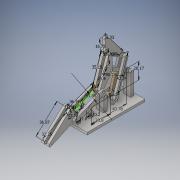
# Autodesk Inventor part: body
Saved by Autodesk Inventor 2016 (Build 200138000, 138)
## iProperties
Created: 2018-05-06
Part Number: body
Material: 一般
Document SubType Name: Modeling
Designer: 黃胤瑋
Density: 1 g/cm^3
Appearance: 預設
Author: 黃胤瑋
Autodesk Inventor part; units mm, degrees
ref_plane "YZ Plane" through (0, 0, 0) normal (1, 0, 0) x (0, 1, 0)
ref_plane "XZ Plane" through (0, 0, 0) normal (0, 1, 0) x (-1, 0, 0)
ref_plane "XY Plane" through (0, 0, 0) normal (0, 0, 1) x (1, 0, 0)
sketch "草圖1" plane through (0, 0, 0) normal (1, 0, 0) x (0, 1, 0)
  line L0 (0, 6) -> (-9.8716, 12.6095)
  line L1 (0, 18.8) -> (-17.0577, 32.3908)
  line L2 (-5.5713, 29.2426) -> (-17.0577, 32.3908)
  line L3 (-5.5713, 29.2426) -> (7.6738, 58.6472)
  line L4 (7.6738, 58.6472) -> (-17.0577, 32.3908)
  line L5 (-19.0401, -5.1652) -> (-52.4584, -16.0617)
  line L6 (-52.4584, -16.0617) -> (-35.2344, -17.5709)
  line L7 (-35.2344, -17.5709) -> (-19.0401, -5.1652)
  line L8 (-52.4584, -16.0617) -> (-69.1174, -14.5223)
  line L9 (-69.1174, -14.5223) -> (-40.2573, -36.5894)
  line L10 (-40.2573, -36.5894) -> (-52.4584, -16.0617)
  line L11 (-40.2573, -36.5894) -> (0, -23.8)
  line L12 (-19.0401, -5.1652) -> (-10.4, -10.2)
  line L13 (-35.2344, -17.5709) -> (-20.17, -43.78)
  line L14 (-19.0401, -5.1652) -> (-9.8716, 12.6095)
  line L15 (-5.5713, 29.2426) -> (-9.8716, 12.6095)
  line L16 (-5.5713, 29.2426) -> (-19.0401, -5.1652)
  point P0 (0, 0)
  dimension "d1" = 11.88
  dimension "d2" = 21.81
  dimension "d3" = 12.8
  dimension "d4" = 36.95
  dimension "d5" = 11.91
  dimension "d6" = 32.25
  dimension "d7" = 36.07
  dimension "d8" = 35.15
  dimension "d9" = 6
  dimension "d10" = 10.2
  dimension "d11" = 10.4
  dimension "d13" = 20.4
  dimension "d14" = 17.29
  dimension "d15" = 23.8
  dimension "d16" = 42.24
  dimension "d18" = 23.88
  dimension "d19" = 36.33
  dimension "d20" = 16.73
  dimension "d22" = 20.17
  dimension "d23" = 43.78
  dimension "d24" = 30.23
  dimension "d25" = 10
  dimension "d26" = 20
  dimension "d105" = 17.18
  constraints: 34 end point, 3 vertical alignment
  measures "d1" distance of L0.start L0.end
  measures "d2" distance of L1.end L1.start
  measures "d3" distance of L0.start L1.start
  measures "d4" distance of L5.start L2.start
  measures "d5" distance of L2.start L1.end
  measures "d6" distance of L2.start L3.end
  measures "d7" distance of L3.end L1.end
  measures "d8" distance of L5.start L5.end
  measures "d9" distance of point (0, 0) L0.start
  measures "d10" vertical distance of point (0, 0) L12.end
  measures "d11" horizontal distance of point (0, 0) L12.end
  measures "d13" distance of L6.end L5.start
  measures "d14" distance of L5.end L6.end
  measures "d15" distance of point (0, 0) L11.end
  measures "d16" distance of L9.end L11.end
  measures "d18" distance of L9.end L5.end
  measures "d19" distance of L8.end L9.end
  measures "d20" distance of L5.end L8.end
  measures "d22" horizontal distance of point (0, 0) L13.end
  measures "d23" vertical distance of point (0, 0) L13.end
  measures "d24" distance of L6.end L13.end
  measures "d25" distance of L5.start L12.end
  measures "d26" distance of L5.start L0.end
  measures "d105" distance of L2.start L0.end
sketch "草圖4" plane through (0, 0, 0) normal (1, 0, 0) x (0, 1, 0)
  line L0 (-53.0784, -14.1602) -> (-19.6601, -3.2637)
  line L1 (-17.8238, -6.7529) -> (-34.0182, -19.1586)
  line L2 (-35.409, -19.5633) -> (-52.633, -18.0541)
  arc A0 (-53.0784, -14.1602) -> (-52.633, -18.0541) centre (-52.4584, -16.0617) ccw
  arc A1 (-35.409, -19.5633) -> (-34.0182, -19.1586) centre (-35.2344, -17.5709) ccw
  arc A2 (-17.8238, -6.7529) -> (-19.6601, -3.2637) centre (-19.0401, -5.1652) ccw
  circle A3 centre (-19.0401, -5.1652) radius 1
  circle A4 centre (-52.4584, -16.0617) radius 1
  circle A5 centre (-35.2344, -17.5709) radius 1
  point P0 (0, 0)
  point P1 (-27.8274, -17.6895)
  dimension "d35" = 2
  dimension "d36" = 2
  dimension "d37" = 2
  dimension "d38" = 2
  constraints: 6 centre point, 6 coincident, 6 end point, 6 point on circle, 6 tangent, 2 equal radius
  measures "d35" radius of A0
  measures "d36" diameter of A3
  measures "d37" diameter of A4
  measures "d38" diameter of A5
extrude "擠出1" add sketch "草圖4" along normal mid plane 3
sketch "草圖5" plane through (-1.5, 0, 0) normal (-1, 0, 0) x (0, 0, 1)
  circle A0 centre (-5.1652, -19.0401) radius 1
  circle A1 centre (-10.2, -10.4) radius 1
  line L0 (-5.1652, -19.0401) -> (-10.2, -10.4) construction
  line L1 (-3.4372, -18.0331) -> (-8.472, -9.393)
  line L2 (-11.928, -11.407) -> (-6.8932, -20.047)
  arc A2 (-6.8932, -20.047) -> (-3.4372, -18.0331) centre (-5.1652, -19.0401) ccw
  arc A3 (-8.472, -9.393) -> (-11.928, -11.407) centre (-10.2, -10.4) ccw
  point P0 (0, 0)
  point P1 (-7.6826, -14.72)
  dimension "d41" = 2
  dimension "d42" = 2
  dimension "d43" = 1
  constraints: 8 end point, 4 centre point, 4 point on circle, 4 tangent, 2 coincident, 1 midpoint, 1 parallel
  measures "d41" diameter of A1
  measures "d42" diameter of A0
  measures "d43" radial gap between concentric circles of A1 A3
extrude "擠出2" add sketch "草圖5" along normal blind 3 separate body
sketch "草圖6" plane through (-1.5, 0, 0) normal (-1, 0, 0) x (0, 0, 1)
  line L0 (-17.5709, -35.2344) -> (-43.78, -20.17) construction
  line L1 (-16.5743, -33.5004) -> (-42.7833, -18.436)
  line L2 (-44.7767, -21.904) -> (-18.5676, -36.9684)
  arc A0 (-18.5676, -36.9684) -> (-16.5743, -33.5004) centre (-17.5709, -35.2344) ccw
  arc A1 (-42.7833, -18.436) -> (-44.7767, -21.904) centre (-43.78, -20.17) ccw
  circle A2 centre (-43.78, -20.17) radius 1
  circle A3 centre (-17.5709, -35.2344) radius 1
  point P0 (0, 0)
  point P1 (-30.6755, -27.7022)
  dimension "d46" = 2
  dimension "d47" = 2
  dimension "d48" = 1
  constraints: 8 end point, 4 centre point, 4 point on circle, 4 tangent, 2 coincident, 1 midpoint, 1 parallel
  measures "d46" diameter of A3
  measures "d47" diameter of A2
  measures "d48" radial gap between concentric circles of A2 A1
extrude "擠出3" add sketch "草圖6" along normal blind 3 separate body
sketch "草圖7" plane through (0, 0, 0) normal (1, 0, 0) x (0, 1, 0)
  circle A0 centre (0, -23.8) radius 1
  circle A1 centre (-40.2573, -36.5894) radius 1
  line L0 (-40.2573, -36.5894) -> (0, -23.8) construction
  line L1 (-40.8628, -34.6833) -> (-0.6056, -21.8939)
  line L2 (0.6056, -25.7061) -> (-39.6517, -38.4955)
  arc A2 (-40.8628, -34.6833) -> (-39.6517, -38.4955) centre (-40.2573, -36.5894) ccw
  arc A3 (0.6056, -25.7061) -> (-0.6056, -21.8939) centre (0, -23.8) ccw
  point P0 (0, 0)
  point P1 (-20.1286, -30.1947)
  dimension "d51" = 2
  dimension "d52" = 2
  dimension "d53" = 1
  constraints: 8 end point, 4 centre point, 4 point on circle, 4 tangent, 2 coincident, 1 midpoint, 1 parallel
  measures "d51" diameter of A0
  measures "d52" diameter of A1
  measures "d53" radial gap between concentric circles of A1 A2
extrude "擠出4" add sketch "草圖7" along normal mid plane 3 separate body
ref_plane "工作平面1" through (-3, 0, 0) normal (-1, 0, 0) x (0, 0, 1)
mirror "鏡射1" about plane through (-3, 0, 0) normal (-1, 0, 0) bodies 1 separate body
sketch "草圖8" plane through (-3, 0, 0) normal (-1, 0, 0) x (0, 0, 1)
  line L0 (-16.111, -70.3323) -> (-38.1782, -41.4721)
  line L1 (-35.5675, -38.538) -> (-15.0398, -50.7392)
  line L2 (-14.0702, -52.2744) -> (-12.5307, -68.9334)
  arc A0 (-16.111, -70.3323) -> (-12.5307, -68.9334) centre (-14.5223, -69.1174) ccw
  arc A1 (-14.0702, -52.2744) -> (-15.0398, -50.7392) centre (-16.0617, -52.4584) ccw
  arc A2 (-35.5675, -38.538) -> (-38.1782, -41.4721) centre (-36.5894, -40.2573) ccw
  circle A3 centre (-14.5223, -69.1174) radius 1
  circle A4 centre (-16.0617, -52.4584) radius 1
  circle A5 centre (-36.5894, -40.2573) radius 1 projected
  circle A6 centre (-36.5894, -40.2573) radius 1
  point P0 (0, 0)
  dimension "d57" = 2
  dimension "d58" = 2
  dimension "d59" = 2
  dimension "d60" = 2
  constraints: 6 centre point, 6 coincident, 6 end point, 6 point on circle, 6 tangent, 2 equal radius
  measures "d57" radius of A0
  measures "d58" diameter of A6
  measures "d59" diameter of A3
  measures "d60" diameter of A4
extrude "擠出5" add sketch "草圖8" along normal mid plane 3 separate body
mirror "鏡射2" about plane through (-3, 0, 0) normal (-1, 0, 0) bodies 4 separate body
sketch "草圖12" plane through (-1.5, 0, 0) normal (-1, 0, 0) x (0, 0, 1)
  circle A0 centre (6, 0) radius 1
  circle A1 centre (12.6095, -9.8716) radius 1
  line L0 (12.6095, -9.8716) -> (6, 0) construction
  line L1 (14.2714, -8.7589) -> (7.6619, 1.1127)
  line L2 (4.3381, -1.1127) -> (10.9476, -10.9843)
  arc A2 (10.9476, -10.9843) -> (14.2714, -8.7589) centre (12.6095, -9.8716) ccw
  arc A3 (7.6619, 1.1127) -> (4.3381, -1.1127) centre (6, 0) ccw
  point P0 (0, 0)
  point P1 (9.3048, -4.9358)
  dimension "d74" = 2
  dimension "d75" = 2
  dimension "d76" = 1
  constraints: 8 end point, 4 centre point, 4 point on circle, 4 tangent, 2 coincident, 1 midpoint, 1 parallel
  measures "d74" diameter of A0
  measures "d75" diameter of A1
  measures "d76" radial gap between concentric circles of A0 A3
extrude "擠出9" add sketch "草圖12" along normal blind 3 separate body
sketch "草圖15" plane through (-1.5, 0, 0) normal (-1, 0, 0) x (0, 0, 1)
  circle A0 centre (18.8, 0) radius 1
  circle A1 centre (32.3908, -17.0577) radius 1
  line L0 (32.3908, -17.0577) -> (18.8, 0) construction
  line L1 (33.955, -15.8114) -> (20.3642, 1.2463)
  line L2 (17.2358, -1.2463) -> (30.8266, -18.304)
  arc A2 (30.8266, -18.304) -> (33.955, -15.8114) centre (32.3908, -17.0577) ccw
  arc A3 (20.3642, 1.2463) -> (17.2358, -1.2463) centre (18.8, 0) ccw
  point P0 (0, 0)
  point P1 (25.5954, -8.5289)
  dimension "d86" = 2
  dimension "d87" = 2
  dimension "d88" = 1
  constraints: 8 end point, 4 centre point, 4 point on circle, 4 tangent, 2 coincident, 1 midpoint, 1 parallel
  measures "d86" diameter of A1
  measures "d87" diameter of A0
  measures "d88" radial gap between concentric circles of A0 A3
extrude "擠出12" add sketch "草圖15" along normal blind 3 separate body
sketch "草圖17" plane through (-1.5, 0, 0) normal (1, 0, 0) x (0, 0, -1)
  line L0 (-33.7621, -18.5136) -> (-60.0185, 6.218)
  line L1 (-57.8258, 9.4974) -> (-28.4212, -3.7478)
  line L2 (-27.3138, -6.1) -> (-30.462, -17.5864)
  arc A0 (-33.7621, -18.5136) -> (-30.462, -17.5864) centre (-32.3908, -17.0577) ccw
  arc A1 (-27.3138, -6.1) -> (-28.4212, -3.7478) centre (-29.2426, -5.5713) ccw
  arc A2 (-57.8258, 9.4974) -> (-60.0185, 6.218) centre (-58.6472, 7.6738) ccw
  circle A3 centre (-32.3908, -17.0577) radius 1 projected
  circle A4 centre (-32.3908, -17.0577) radius 1
  circle A5 centre (-29.2426, -5.5713) radius 1
  circle A6 centre (-58.6472, 7.6738) radius 1
  point P0 (0, 0)
  dimension "d97" = 2
  dimension "d98" = 2
  dimension "d99" = 2
  dimension "d100" = 2
  constraints: 6 centre point, 6 coincident, 6 end point, 6 point on circle, 6 tangent, 2 equal radius
  measures "d97" radius of A0
  measures "d98" diameter of A6
  measures "d99" diameter of A5
  measures "d100" diameter of A4
extrude "擠出14" add sketch "草圖17" along normal blind 3 separate body
mirror "鏡射3" about plane through (-3, 0, 0) normal (-1, 0, 0) bodies 10 separate body
sketch "草圖19" plane through (1.5, 0, 0) normal (1, 0, 0) x (0, 0, -1)
  line L0 (4.4361, -20.9024) -> (-29.9716, -7.4337)
  line L1 (-28.742, -3.635) -> (-12.1089, -7.9353)
  line L2 (-11.6927, -8.0941) -> (6.082, -17.2626)
  arc A0 (4.4361, -20.9024) -> (6.082, -17.2626) centre (5.1652, -19.0401) ccw
  arc A1 (-28.742, -3.635) -> (-29.9716, -7.4337) centre (-29.2426, -5.5713) ccw
  arc A2 (-11.6927, -8.0941) -> (-12.1089, -7.9353) centre (-12.6095, -9.8716) ccw
  circle A3 centre (-12.6095, -9.8716) radius 1
  circle A4 centre (5.1652, -19.0401) radius 1 projected
  circle A5 centre (5.1652, -19.0401) radius 1
  circle A6 centre (-29.2426, -5.5713) radius 1 projected
  circle A7 centre (-29.2426, -5.5713) radius 1
  dimension "d107" = 2
  dimension "d108" = 2
  dimension "d109" = 2
  constraints: 6 centre point, 6 end point, 6 point on circle, 6 tangent, 5 coincident, 1 equal radius
  measures "d107" radius of A0
  measures "d108" radius of A2
  measures "d109" diameter of A3
extrude "擠出16" add sketch "草圖19" along normal blind 3 separate body
mirror "鏡射4" about plane through (-3, 0, 0) normal (-1, 0, 0) bodies 12 separate body
move or copy body "移動本體1" bodies to move or copy 8 copy no translate (-3, 0, 0)
mirror "鏡射5" about plane through (-3, 0, 0) normal (-1, 0, 0) bodies 8 separate body
sketch "草圖22" plane through (-3, 0, 0) normal (-1, 0, 0) x (0, 0, 1)
  circle A0 centre (6, 0) radius 2
  circle A1 centre (-23.8, 0) radius 1 projected
  circle A2 centre (-23.8, 0) radius 2
  point P0 (0, 0)
  point P1 (18.8, 0)
  dimension "d117" = 4
  dimension "d118" = 4
  constraints: 2 centre point, 2 coincident
  measures "d117" diameter of A0
  measures "d118" diameter of A2
extrude "擠出18" add sketch "草圖22" along normal mid plane 3 separate body
sketch "草圖24" plane through (-3, 0, 0) normal (-1, 0, 0) x (0, 0, 1)
  circle A0 centre (6, 0) radius 2 projected
  circle A1 centre (-23.8, 0) radius 2 projected
  line L0 (6, 0) -> (4, 0)
  line L1 (4.5, 6.3553) -> (6, 6.3553)
  line L2 (6, 6.3553) -> (6, 0)
  line L3 (4.5, 0) -> (4.5, 6.3553)
  point P0 (0, 0)
  dimension "d159" = 3
  constraints: 8 end point, 1 horizontal, 1 horizontal alignment, 1 parallel, 1 perpendicular, 1 point on line, 1 other
  measures "d159" diameter of L3 L2
revolve "迴轉1" add sketch "草圖24" angle 360 about axis through (-3, 6.3553, 6) along (0, -1, 0) bodies 15 contours L3 L1 L2 A0 | A0 L2 L0 L3
sketch "草圖25" plane through (-3, 0, 0) normal (-1, 0, 0) x (0, 0, 1)
  circle A0 centre (-23.8, 0) radius 2 projected
  line L0 (-23.8, 0) -> (-25.3, 0)
  line L1 (-25.3, 6.3553) -> (-23.8, 6.3553)
  line L2 (-23.8, 6.3553) -> (-23.8, 0)
  line L3 (7.5, 6.3553) -> (4.5, 6.3553) projected
  line L4 (-25.3, 0) -> (-25.3, 6.3553)
  point P0 (0, 0)
  point P1 (-25.8, 0)
  dimension "d160" = 3
  constraints: 8 end point, 2 horizontal alignment, 1 horizontal, 1 parallel, 1 perpendicular, 1 other
  measures "d160" diameter of L4 L2
revolve "迴轉2" add sketch "草圖25" angle 360 about axis through (-3, 6.3553, -23.8) along (0, -1, 0) picked at (-24.8, 0.441) bodies 15 contours L2 L0 L4 A0 | A0 L4 L1 L2
sketch "草圖30" plane through (-3, 0, 0) normal (-1, 0, 0) x (0, 0, 1)
  circle A0 centre (-10.2, -10.4) radius 1 projected
  circle A1 centre (-5.1652, -19.0401) radius 1 projected
  line L0 (-3.4372, -18.0331) -> (-8.472, -9.393) projected
  arc A2 (-8.472, -9.393) -> (-11.928, -11.407) centre (-10.2, -10.4) ccw projected
  line L1 (-11.928, -11.407) -> (-6.8932, -20.047) projected
  arc A3 (-6.8932, -20.047) -> (-3.4372, -18.0331) centre (-5.1652, -19.0401) ccw projected
  circle A4 centre (-10.2, -10.4) radius 2
  line L2 (-8.2, -10.4) -> (-12.2, -10.4)
  line L3 (-12.2, -10.4) -> (-12.2, 6.3553)
  line L4 (-12.2, 6.3553) -> (-8.2, 6.3553)
  line L5 (-8.2, 6.3553) -> (-8.2, -10.4)
  line L6 (7.5, 6.3553) -> (4.5, 6.3553) projected
  point P0 (0, 0)
  constraints: 8 end point, 3 point on circle, 2 horizontal alignment, 2 parallel, 1 centre point, 1 coincident, 1 horizontal, 1 perpendicular
extrude "擠出23" add sketch "草圖30" along normal mid plane 9 contours L2 A4 A2 A0 | A0 L2 A2 A4 | A4 L0 L5 | L3 L4 L5 L0 A2 bodies 15
sketch "草圖31" plane through (-7.5, 0, 0) normal (-1, 0, 0) x (0, 0, 1)
  line L0 (-9.2, -10.4) -> (-11.2, -10.4) projected
  arc A0 (-11.2, -10.4) -> (-9.2, -10.4) centre (-10.2, -10.4) ccw projected
  arc A1 (-12.2, -10.4) -> (-8.2, -10.4) centre (-10.2, -10.4) ccw projected
  line L1 (-8.2, -10.4) -> (-8.2, 6.3553) projected
  line L2 (-8.2, 6.3553) -> (-12.2, 6.3553) projected
  line L3 (-12.2, 6.3553) -> (-12.2, -10.4) projected
  circle A2 centre (-10.2, -10.4) radius 1
  point P0 (0, 0)
  constraints: 1 coincident, 1 horizontal alignment, 2 other
extrude "擠出24" cut sketch "草圖31" against normal blind 9 contours L0 A2 bodies 3 15
sketch "草圖32" plane through (-3, 0, 0) normal (-1, 0, 0) x (0, 0, 1)
  arc A0 (-12.2, -10.4) -> (-8.2, -10.4) centre (-10.2, -10.4) ccw projected
  line L0 (-12.2, -10.4) -> (-12.2, 6.3553) projected
  line L1 (-12.2, 6.3553) -> (-8.2, 6.3553) projected
  line L2 (-8.2, 6.3553) -> (-8.2, -10.4) projected
  circle A1 centre (-10.2, -10.4) radius 1 projected
  line L3 (-8.2, -8.4) -> (-12.2, -8.4)
  line L4 (-12.2, -10.4) -> (-12.2, 6.3553) projected
  circle A2 centre (-10.2, -10.4) radius 2
  line L5 (-8.2, -8.4) -> (-8.2, -10.4)
  line L6 (-12.2, -8.4) -> (-12.2, -10.4)
  point P0 (0, 0)
  constraints: 6 end point, 5 point on circle, 3 tangent, 2 point on line, 1 centre point, 1 coincident, 1 horizontal
extrude "擠出25" cut sketch "草圖32" along normal mid plane 3 contours A2 A0 | L0 L3 A2 | A2 L3 L2 bodies 3 15
sketch "草圖33" plane through (-4.5, 0, 0) normal (-1, 0, 0) x (0, 0, 1)
  arc A0 (-42.7833, -18.436) -> (-44.7767, -21.904) centre (-43.78, -20.17) ccw projected
  circle A1 centre (-43.78, -20.17) radius 2
  line L0 (-41.78, -20.17) -> (-45.78, -20.17)
  line L1 (-45.78, -20.17) -> (-45.78, 6.3553)
  line L2 (-45.78, 6.3553) -> (-41.78, 6.3553)
  line L3 (-41.78, 6.3553) -> (-41.78, -20.17)
  line L4 (-22.3, 6.3553) -> (-25.3, 6.3553) projected
  point P0 (0, 0)
  constraints: 8 end point, 3 point on circle, 2 horizontal alignment, 2 parallel, 1 centre point, 1 coincident, 1 horizontal, 1 perpendicular
extrude "擠出26" add sketch "草圖33" along normal blind 3 and the other way blind 6 bodies 15
sketch "草圖34" plane through (-7.5, 0, 0) normal (-1, 0, 0) x (0, 0, 1)
  arc A0 (-45.78, -20.17) -> (-41.78, -20.17) centre (-43.78, -20.17) ccw projected
  line L0 (-41.78, -20.17) -> (-41.78, 6.3553) projected
  line L1 (-41.78, 6.3553) -> (-45.78, 6.3553) projected
  line L2 (-45.78, 6.3553) -> (-45.78, -20.17) projected
  circle A1 centre (-43.78, -20.17) radius 1
  point P0 (0, 0)
  dimension "d142" = 2
  constraints: 1 centre point, 1 coincident
  measures "d142" diameter of A1
extrude "擠出27" cut sketch "草圖34" against normal through all contours A1 bodies 3 15
sketch "草圖35" plane through (-3, 0, 0) normal (-1, 0, 0) x (0, 0, 1)
  circle A0 centre (-43.78, -20.17) radius 1 projected
  arc A1 (-45.78, -20.17) -> (-41.78, -20.17) centre (-43.78, -20.17) ccw projected
  line L0 (-45.78, -20.17) -> (-45.78, 6.3553) projected
  line L1 (-45.78, 6.3553) -> (-41.78, 6.3553) projected
  line L2 (-41.78, 6.3553) -> (-41.78, -20.17) projected
  circle A2 centre (-43.78, -20.17) radius 2
  line L3 (-41.78, -18.17) -> (-45.78, -18.17)
  line L4 (-45.78, -18.17) -> (-45.78, -20.17)
  line L5 (-41.78, -18.17) -> (-41.78, -20.17)
  point P0 (0, 0)
  constraints: 6 end point, 4 point on circle, 3 tangent, 2 point on line, 1 centre point, 1 coincident, 1 concentric, 1 perpendicular
extrude "擠出28" cut sketch "草圖35" along normal mid plane 3 contours A2 A1 | L0 L3 A2 | A2 L3 L2 bodies 15
sketch "草圖36" plane through (-7.5, 6.3553, -12.2) normal (0, 1, 0) x (1, 0, 0)
  line L0 (-10.5, -35.4) -> (19.5, -35.4)
  line L1 (19.5, -35.4) -> (19.5, 36.6)
  line L2 (19.5, 36.6) -> (-10.5, 36.6)
  line L3 (-10.5, 36.6) -> (-10.5, -35.4)
  circle A0 centre (4.5, 11.6) radius 1.5 projected
  point P0 (7.5, -12.2)
  dimension "d147" = 30
  dimension "d148" = 15
  dimension "d149" = 72
  dimension "d150" = 25
  constraints: 8 end point, 2 parallel, 1 horizontal, 1 perpendicular
  measures "d147" distance of L1.end L2.end
  measures "d148" distance from line of L3 A0.centre
  measures "d149" distance of L2.end L0.start
  measures "d150" distance from line of A0.centre L2
extrude "擠出29" add sketch "草圖36" along normal blind 3 contours L3 L2 L1 L0 | A0 bodies 15
sketch "草圖37" plane through (-3, 0, 0) normal (-1, 0, 0) x (0, 0, 1)
  circle A0 centre (6, 0) radius 1 projected
  circle A1 centre (-23.8, 0) radius 1 projected
  point P0 (0, 0)
extrude "擠出30" cut sketch "草圖37" against normal through all bodies 3 15
sketch "草圖38" plane through (-7.5, -40.8628, -34.6833) normal (-1, 0, 0) x (0, -0.3027797, 0.9530606)
  circle A0 centre (-2, 42.24) radius 1 projected
  point P0 (20.6828, 49.4462)
extrude "擠出31" cut sketch "草圖38" against normal blind 30 bodies 7 15
sketch "草圖39" plane through (-7.5, -8.7589, 14.2714) normal (-1, 0, 0) x (0, 0.5563569, 0.8309434)
  circle A0 centre (-2, 11.88) radius 1 projected
  point P0 (-6.9857, 15.2181)
extrude "擠出32" cut sketch "草圖39" against normal blind 30 bodies 15
sketch "草圖40" plane through (-3, 0, 0) normal (-1, 0, 0) x (0, 0, 1)
  arc A0 (20.3642, 1.2463) -> (17.2358, -1.2463) centre (18.8, 0) ccw projected
  circle A1 centre (18.8, 0) radius 2
  line L0 (19.2218, -3.7389) -> (22.3502, -1.2463)
  line L1 (33.955, -15.8114) -> (20.3642, 1.2463) projected
  line L2 (17.2358, -1.2463) -> (30.8266, -18.304) projected
  point P0 (0, 0)
  dimension "d161" = 90
  constraints: 2 end point, 2 point on line, 1 coincident, 3 other
  measures "d161" angle of L1 L0
extrude "擠出33" cut sketch "草圖40" along normal mid plane 1.5 bodies 3 9
sketch "草圖41" plane through (-3, 0, 0) normal (-1, 0, 0) x (0, 0, 1)
  arc A0 (20.3642, 1.2463) -> (17.2358, -1.2463) centre (18.8, 0) ccw projected
  arc A1 (16.8, 0) -> (20.8, 0) centre (18.8, 0) ccw
  line L0 (16.8, 0) -> (16.8, 7.1661)
  line L1 (16.8, 7.1661) -> (20.8, 7.1661)
  line L2 (20.8, 7.1661) -> (20.8, 0)
  line L3 (23.2, 6.3553) -> (-48.8, 6.3553) projected
  circle A2 centre (18.8, 0) radius 1 projected
  point P0 (0, 0)
  constraints: 6 end point, 3 point on circle, 1 centre point, 1 coincident, 1 concentric, 1 parallel
extrude "擠出34" add sketch "草圖41" along normal mid plane 1.5 bodies 15
